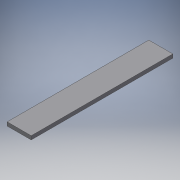
# Autodesk Inventor part: LIghtTile_new
Saved by Autodesk Inventor 2017 (Build 210142000, 142)
## iProperties
Created: 2017-05-28
Part Number: LIghtTile_new
Material: Generic
Document SubType Name: Modeling
Designer: Paolo
Density: 1 g/cm^3
Appearance: Default
Author: Paolo
Autodesk Inventor part; units mm, degrees
ref_plane "YZ Plane" through (0, 0, 0) normal (1, 0, 0) x (0, 1, 0)
ref_plane "XZ Plane" through (0, 0, 0) normal (0, 1, 0) x (-1, 0, 0)
ref_plane "XY Plane" through (0, 0, 0) normal (0, 0, 1) x (1, 0, 0)
sketch "Sketch1" plane through (0, 0, 0) normal (0, 0, 1) x (1, 0, 0)
  line L0 (-10, 57) -> (10, 57) projected
  line L1 (-10, 55) -> (-10, 57) projected
  line L2 (-10, 55) -> (10, 55) projected
  line L3 (10, 55) -> (10, 57) projected
  line L4 (-10, -57) -> (-10, -59) projected
  line L5 (-10, -59) -> (10, -59) projected
  line L6 (10, -57) -> (10, -59) projected
  line L7 (-10, -57) -> (10, -57) projected
  line L8 (9.8, 55.2) -> (-9.8, 55.2)
  line L9 (-9.8, 55.2) -> (-9.8, 56.8)
  line L10 (-9.8, 56.8) -> (9.8, 56.8)
  line L11 (9.8, 56.8) -> (9.8, 55.2)
  line L12 (9.8, -58.8) -> (-9.8, -58.8)
  line L13 (-9.8, -58.8) -> (-9.8, -57.2)
  line L14 (-9.8, -57.2) -> (9.8, -57.2)
  line L15 (9.8, -57.2) -> (9.8, -58.8)
  line L16 (-9.8, 55.2) -> (9.8, 55.2)
  line L17 (9.8, 55.2) -> (9.8, -57.2)
  line L18 (9.8, -57.2) -> (-9.8, -57.2)
  line L19 (-9.8, -57.2) -> (-9.8, 55.2)
  point P0 (0, 0)
  dimension "d0" = 0.2
  dimension "d1" = 0.2
  constraints: 24 end point, 2 parallel, 1 horizontal, 1 perpendicular, 6 other
  measures "d0" distance between parallel lines of L2 L8
  measures "d1" distance between parallel lines of L5 L12
extrude "Extrusion1" add sketch "Sketch1" along normal blind 3 contours L19 L8 L17 L2 | L2 L17 L7 L19 | L7 L17 L14 L19 | L9 L10 L11 L8 | L14 L15 L12 L13
body "Solid1"
